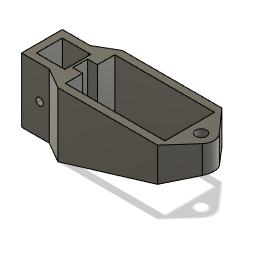
Soporte Servo + Eje en Perfil 10x10 v6 (Autodesk Fusion 360 design; units mm, degrees)
Autodesk Fusion 360 part; units mm, degrees
sketch "Boceto1" plane through (0, 0, 0) normal (0, 1, 0) x (1, 0, 0)
  line L0 (425.7705, -21.5897) -> (436.2705, -21.5897)
  line L1 (436.2705, -21.5897) -> (436.2705, -32.0897)
  line L2 (436.2705, -32.0897) -> (425.7705, -32.0897)
  line L3 (425.7705, -32.0897) -> (425.7705, -21.5897)
  line L4 (422.7705, -18.5897) -> (434, -18.5897)
  line L5 (434, -35.0897) -> (422.7705, -35.0897)
  line L6 (422.7705, -35.0897) -> (422.7705, -18.5897)
  line L7 (442.2705, -16.8147) -> (482.6205, -16.8147)
  line L8 (482.6205, -16.8147) -> (482.6205, -36.8647)
  line L9 (482.6205, -36.8647) -> (442.2705, -36.8647)
  line L10 (442.2705, -36.8647) -> (442.2705, -16.8147)
  line L11 (482.6205, -13.8147) -> (482.6205, -39.8647)
  line L12 (437.2705, -26.8397) -> (442.2705, -26.8397)
  circle A0 centre (487.2705, -26.8397) radius 2.2
  line L13 (482.6205, -26.8397) -> (485.0705, -26.8397)
  line L14 (485.0705, -26.8397) -> (487.2705, -26.8397)
  circle A1 centre (487.2705, -26.8397) radius 5.2
  line L15 (425.7705, -21.5897) -> (425.7705, -18.5897)
  line L16 (425.7705, -21.5897) -> (422.7705, -21.5897)
  line L17 (425.7705, -32.0897) -> (425.7705, -35.0897)
  line L18 (442.2705, -23.8397) -> (438.2705, -23.8397)
  line L19 (438.2705, -23.8397) -> (438.2705, -29.8397)
  line L20 (438.2705, -29.8397) -> (442.2705, -29.8397)
  line L21 (442.2705, -29.8397) -> (442.2705, -23.8397)
  line L22 (482.6205, -13.8147) -> (491.1511, -23.3783)
  line L23 (482.6205, -39.8647) -> (491.1511, -30.3011)
  line L24 (442.2705, -16.8147) -> (442.2705, -13.8147)
  line L25 (442.2705, -36.8647) -> (442.2705, -39.8647)
  line L26 (434, -18.5897) -> (442.2705, -13.8147)
  line L27 (482.6205, -13.8147) -> (442.2705, -13.8147)
  line L28 (434, -35.0897) -> (442.2705, -39.8647)
  line L29 (482.6205, -39.8647) -> (442.2705, -39.8647)
  line L30 (437.2705, -26.8397) -> (436.2705, -26.8397)
  line L31 (436.2705, -32.0897) -> (437.2705, -32.0897)
  line L32 (436.2705, -21.5897) -> (437.2705, -21.5897)
  line L33 (434, -18.5897) -> (437.2705, -21.5897)
  line L34 (437.2705, -21.5897) -> (437.2705, -26.8397)
  line L35 (437.2705, -26.8397) -> (437.2705, -32.0897)
  line L36 (437.2705, -32.0897) -> (434, -35.0897)
  point P0 (438.2705, -26.8397)
  dimension "d2" = 10.5
  dimension "d3" = 3
  dimension "d7" = 40.35
  dimension "d8" = 20.05
  dimension "d12" = 4.4
  dimension "d14" = 48.8
  dimension "d15" = 3
  dimension "d16" = 3
  dimension "d17" = 4
  dimension "d18" = 6
  dimension "d29" = 3
  dimension "d73" = 1
  dimension "d74" = 5
  dimension "d75" = 150
  constraint horizontal L0
  constraint vertical L1
  constraint horizontal L2
  constraint vertical L3
  constraint horizontal L4
  constraint horizontal L5
  constraint vertical L6
  constraint horizontal L7
  constraint vertical L8
  constraint horizontal L9
  constraint vertical L10
  constraint vertical L11
  constraint coincident L10 L12.end
  constraint perpendicular L10 L12
  constraint midpoint L10 L12.end
  constraint coincident L11 L13.start
  constraint coincident A0 L13.end
  constraint perpendicular L11 L13
  constraint coincident A0.centre L14.end
  constraint coincident L4 L15.end
  constraint perpendicular L4 L15
  constraint coincident L6 L16.end
  constraint perpendicular L6 L16
  constraint coincident L5 L17.end
  constraint perpendicular L5 L17
  constraint equal L15 L17
  constraint equal L0 L3
  constraint horizontal L18
  constraint vertical L19
  constraint horizontal L20
  constraint vertical L21
  constraint coincident L10 L18.start
  constraint coincident L19 P0
  constraint coincident L12 P0
  constraint midpoint L19 P0
  constraint parallel L13 L14
  constraint coincident A1 L22.end
  constraint tangent A1 L22
  constraint coincident A1 L23.end
  constraint tangent A1 L23
  constraint midpoint L8 L11
  constraint vertical L24
  constraint horizontal L27
  constraint equal L24 L25
  constraint vertical L25
  constraint midpoint L8 L13.start
  constraint midpoint L1 L30.end
  constraint perpendicular L1 L30
  constraint perpendicular L1 L32
  constraint equal L30 L32
  constraint equal L30 L31
  constraint perpendicular L31 L35
  constraint vertical L5.start L4.end
  measures "d2" distance of L0.start L0.end
  measures "d3" distance of L0 L4
  measures "d7" distance of L7.start L7.end
  measures "d8" distance of L7.start L9.end
  measures "d12" diameter of A0
  measures "d14" distance of L1 L13.end
  measures "d15" distance of A0 A1
  measures "d16" distance of L6 L15
  measures "d17" distance of L18.start L18.end
  measures "d18" distance of L18.end L19.end
  measures "d29" distance of L7.start L24.end
  measures "d73" distance of L12.start L30.end
  measures "d74" distance of L12.start L12.end
  measures "d75" angle of L4 L26
extrude "Extruir2" add sketch "Boceto1" along normal blind 26 contours L0 L4 L15 L32 L33 | L4 L6 L15 L16 | L3 L5 L6 L16 L17 | L2 L5 L17 L31 L36 | L10 L12 L18 L19 L24 L26 L33 L34 | L10 L12 L19 L20 L25 L28 L35 L36 | L7 L11 L24 L27 | L9 L11 L25 L29 | L8 L11 A1 L22 | L8 L11 A1 L23 | L8 L11 A1 picked at (483.4698, -25.8477)
hole "Agujero2" at (430.1152, 12.5894, 35.0897) direction (0, 0, -1) diameter 3 depth 20 tip angle 180
sketch "Boceto6" plane through (0, 0, 13.8147) normal (0, 0, -1) x (-1, 0, 0)
  line L0 (-482.6205, 0) -> (-442.2705, 0)
  line L1 (-442.2705, 0) -> (-442.2705, 26)
  line L2 (-442.2705, 26) -> (-482.6205, 26)
  line L3 (-482.6205, 26) -> (-482.6205, 0)
  line L4 (-495, 0) -> (-442.2705, 0)
  line L5 (-442.2705, 0) -> (-495, 16)
  line L6 (-495, 16) -> (-495, 0)
  constraint coincident L0.end L1.start
  constraint perpendicular L4 L6
extrude "Extruir11" cut sketch "Boceto6" against normal blind 30 contours L0 L3 L4 L5 | L3 L4 L5 L6
